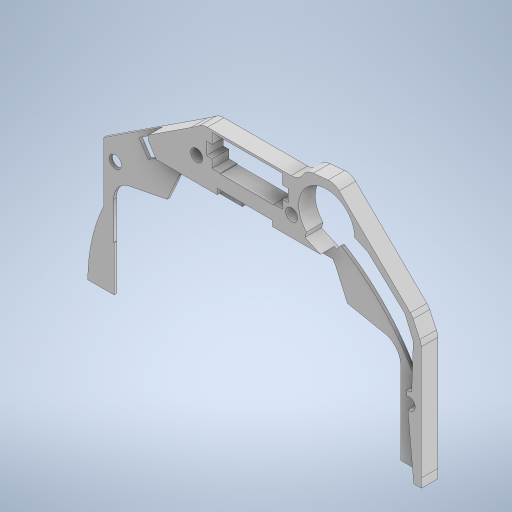
# Autodesk Inventor part: separator_right
Saved by Autodesk Inventor 2023.4 (Build 274418000, 418)
## iProperties
Created: 2024-02-02
Part Number: separator_right
Material: Generic
Document SubType Name: Modeling
Designer: aaron
Density: 1 g/cm^3
Appearance: Default
Author: aaron
Autodesk Inventor part; units mm, degrees
ref_plane "YZ Plane" through (0, 0, 0) normal (1, 0, 0) x (0, 1, 0)
ref_plane "XZ Plane" through (0, 0, 0) normal (0, 1, 0) x (-1, 0, 0)
ref_plane "XY Plane" through (0, 0, 0) normal (0, 0, 1) x (1, 0, 0)
sketch "Sketch1" plane through (0, 0, 0) normal (0, 0, 1) x (1, 0, 0)
  circle A0 centre (17.4431, 31.8315) radius 2.15
  circle A1 centre (-16.9982, 33.272) radius 2.15
  circle A2 centre (60.1072, -6.2422) radius 2.15
  circle A3 centre (-51.4779, 11.4956) radius 2.15
  arc A4 (-55.7008, -4.5478) -> (-61.4978, -30.6135) centre (0.0022, -30.6135) ccw
  line L0 (-61.4978, -30.6135) -> (-51.9975, -30.6135)
  line L1 (-51.9975, -30.6135) -> (-51.9975, -14.2185)
  line L2 (-51.9975, -14.2185) -> (-52.0975, -14.2185)
  line L3 (-52.0975, -14.2185) -> (-52.0975, -0.6135)
  arc A5 (-46.3779, 6.351) -> (-52.0975, -0.6135) centre (-44.9975, -0.6135) ccw
  line L4 (-46.3779, 6.351) -> (-32.7026, 9.0616)
  line L5 (-32.7026, 9.0616) -> (-28.4427, 18.6544)
  line L6 (-28.4427, 18.6544) -> (-27.4427, 20.3865)
  line L7 (-27.4427, 20.3865) -> (-5.4427, 20.3865)
  line L8 (-5.4427, 20.3865) -> (-5.4427, 23.8865)
  line L9 (-4.9427, 24.3865) -> (-5.4427, 23.8865)
  line L10 (-4.9427, 24.3865) -> (6.0573, 24.3865)
  line L11 (6.5573, 23.8865) -> (6.0573, 24.3865)
  line L12 (6.5573, 23.8865) -> (6.5573, 20.3865)
  line L13 (6.5573, 20.3865) -> (27.4471, 20.3865)
  line L14 (27.4471, 20.3865) -> (28.4471, 18.6544)
  line L15 (28.4471, 18.6544) -> (32.707, 9.0616)
  line L16 (32.707, 9.0616) -> (46.3823, 6.351)
  arc A6 (49.1747, 5.1308) -> (46.3823, 6.351) centre (45.0019, -0.6135) ccw
  line L17 (49.1747, 5.1308) -> (49.1159, 5.0499)
  arc A7 (52.0019, -0.6135) -> (49.1159, 5.0499) centre (45.0019, -0.6135) ccw
  line L18 (52.0019, -0.6135) -> (52.0019, -30.6135)
  line L19 (52.0019, -30.6135) -> (64.5022, -30.6135)
  arc A8 (64.5022, -30.6135) -> (64.4236, -27.4299) centre (0.0022, -30.6135) ccw
  line L20 (64.4236, -27.4299) -> (64.4236, 13.7348)
  arc A9 (64.4236, 13.7348) -> (63.951, 15.8567) centre (59.4236, 13.7348) ccw
  line L21 (63.951, 15.8567) -> (61.5154, 21.0535)
  arc A10 (61.5154, 21.0535) -> (60.4923, 22.4981) centre (56.988, 18.9315) ccw
  line L22 (60.4923, 22.4981) -> (34.6486, 47.8907)
  arc A11 (34.6486, 47.8907) -> (30.6723, 49.3019) centre (31.1444, 44.3242) ccw
  line L23 (30.6723, 49.3019) -> (25.3285, 48.7951)
  arc A12 (25.3285, 48.7951) -> (21.5187, 46.3993) centre (25.8005, 43.8174) ccw
  arc A13 (17.237, 43.9813) -> (21.5187, 46.3993) centre (17.237, 48.9813) ccw
  line L24 (-13.1205, 43.9813) -> (17.237, 43.9813)
  arc A14 (-13.1205, 43.9813) -> (-15.9723, 43.0882) centre (-13.1205, 38.9813) ccw
  line L25 (-15.9723, 43.0882) -> (-19.2592, 40.8057)
  line L26 (-55.7008, 17.024) -> (-19.2592, 40.8057)
  line L27 (-55.7008, -4.5478) -> (-55.7008, 17.024)
  line L28 (-8.3739, 31.6813) -> (-8.3739, 31.9813)
  line L29 (-8.3739, 31.9813) -> (-11.3739, 31.9813)
  line L30 (-11.3739, 31.9813) -> (-11.3739, 34.9813)
  line L31 (-11.3739, 34.9813) -> (-13.3739, 34.9813)
  line L32 (-13.3739, 34.9813) -> (-13.3739, 39.4813)
  line L33 (-13.3739, 39.4813) -> (-11.3739, 39.4813)
  line L34 (-11.3739, 39.4813) -> (-11.3739, 43.1813)
  line L35 (-11.3739, 43.1813) -> (14.1261, 43.1813)
  line L36 (14.1261, 43.1813) -> (14.1261, 39.4813)
  line L37 (14.1261, 39.4813) -> (16.1261, 39.4813)
  line L38 (16.1261, 39.4813) -> (16.1261, 34.9813)
  line L39 (16.1261, 34.9813) -> (14.1261, 34.9813)
  line L40 (14.1261, 34.9813) -> (14.1261, 31.9813)
  line L41 (14.1261, 31.9813) -> (11.1261, 31.9813)
  line L42 (11.1261, 31.9813) -> (11.1261, 31.6813)
  line L43 (11.1261, 31.6813) -> (-8.3739, 31.6813)
  arc A15 (30.18, 25.9182) -> (30.7743, 25.9371) centre (30.1536, 36.0569) ccw
  line L44 (30.18, 25.9182) -> (28.8398, 24.1662)
  line L45 (28.8398, 24.1662) -> (22.2728, 27.0821)
  line L46 (22.2728, 27.0821) -> (22.8312, 29.0443)
  arc A16 (40.2924, 36.0753) -> (22.8312, 29.0443) centre (30.1536, 36.0569) ccw
  line L47 (40.2924, 36.0753) -> (45.0482, 33.9636)
  line L48 (45.0482, 33.9636) -> (58.5651, 21.2864)
  line L49 (58.5651, 21.2864) -> (61.5673, 14.035)
  line L50 (61.5673, 14.035) -> (61.0022, -2.0891)
  line L51 (61.0022, -2.0891) -> (57.5886, -2.9772)
  arc A17 (57.5886, -2.9772) -> (30.7743, 25.9371) centre (-6.906, -35.8969) ccw
  line L52 (-39.547, 18.1923) -> (-42.9354, 23.3844)
  line L53 (-34.4498, 28.9221) -> (-42.9354, 23.3844)
  line L54 (-34.4498, 28.9221) -> (-31.0613, 23.73)
  line L55 (-31.0613, 23.73) -> (-39.547, 18.1923)
  point P0 (0, 0)
  constraints: 112 end point, 28 point on circle, 18 centre point
extrude "Extrusion1" add sketch "Sketch1" along normal blind 1
sketch "Sketch2" plane through (0, 0, 1) normal (0, 0, 1) x (1, 0, 0)
  line L0 (-19.2592, 40.8057) -> (-55.7008, 17.024) projected
  line L1 (-55.7008, 17.024) -> (-55.7008, -4.5478) projected
  arc A0 (-55.7008, -4.5478) -> (-61.4978, -30.6135) centre (0.0022, -30.6135) ccw projected
  line L2 (-61.4978, -30.6135) -> (-51.9975, -30.6135) projected
  line L3 (-51.9975, -30.6135) -> (-51.9975, -14.2185) projected
  line L4 (-51.9975, -14.2185) -> (-52.0975, -14.2185) projected
  line L5 (-52.0975, -14.2185) -> (-52.0975, -0.6135) projected
  arc A1 (-46.3779, 6.351) -> (-52.0975, -0.6135) centre (-44.9975, -0.6135) ccw projected
  line L6 (-46.3779, 6.351) -> (-32.7026, 9.0616) projected
  line L7 (-32.7026, 9.0616) -> (-28.4427, 18.6544) projected
  line L8 (-28.4427, 18.6544) -> (-27.4427, 20.3865) projected
  line L9 (-27.4427, 20.3865) -> (-5.4427, 20.3865) projected
  line L10 (-5.4427, 20.3865) -> (-5.4427, 23.8865) projected
  line L11 (-5.4427, 23.8865) -> (-4.9427, 24.3865) projected
  line L12 (-4.9427, 24.3865) -> (6.0573, 24.3865) projected
  line L13 (6.0573, 24.3865) -> (6.5573, 23.8865) projected
  line L14 (6.5573, 23.8865) -> (6.5573, 20.3865) projected
  line L15 (6.5573, 20.3865) -> (27.4471, 20.3865) projected
  line L16 (27.4471, 20.3865) -> (28.4471, 18.6544) projected
  line L17 (28.4471, 18.6544) -> (32.707, 9.0616) projected
  line L18 (32.707, 9.0616) -> (46.3823, 6.351) projected
  arc A2 (49.1747, 5.1308) -> (46.3823, 6.351) centre (45.0019, -0.6135) ccw projected
  line L19 (49.1747, 5.1308) -> (49.1159, 5.0499) projected
  arc A3 (52.0019, -0.6135) -> (49.1159, 5.0499) centre (45.0019, -0.6135) ccw projected
  line L20 (52.0019, -0.6135) -> (52.0019, -30.6135) projected
  line L21 (52.0019, -30.6135) -> (64.5022, -30.6135) projected
  arc A4 (64.5022, -30.6135) -> (64.4236, -27.4299) centre (0.0022, -30.6135) ccw projected
  line L22 (64.4236, -27.4299) -> (64.4236, 13.7348) projected
  arc A5 (64.4236, 13.7348) -> (63.951, 15.8567) centre (59.4236, 13.7348) ccw projected
  line L23 (63.951, 15.8567) -> (61.5154, 21.0535) projected
  arc A6 (61.5154, 21.0535) -> (60.4923, 22.4981) centre (56.988, 18.9315) ccw projected
  line L24 (60.4923, 22.4981) -> (34.6486, 47.8907) projected
  arc A7 (34.6486, 47.8907) -> (30.6723, 49.3019) centre (31.1444, 44.3242) ccw projected
  line L25 (30.6723, 49.3019) -> (25.3285, 48.7951) projected
  arc A8 (25.3285, 48.7951) -> (21.5187, 46.3993) centre (25.8005, 43.8174) ccw projected
  arc A9 (17.237, 43.9813) -> (21.5187, 46.3993) centre (17.237, 48.9813) ccw projected
  line L26 (17.237, 43.9813) -> (-13.1205, 43.9813) projected
  arc A10 (-13.1205, 43.9813) -> (-15.9723, 43.0882) centre (-13.1205, 38.9813) ccw projected
  line L27 (-15.9723, 43.0882) -> (-19.2592, 40.8057) projected
  circle A11 centre (60.1072, -6.2422) radius 2.15 projected
  circle A12 centre (-51.4779, 11.4956) radius 2.15 projected
  circle A13 centre (17.4431, 31.8315) radius 2.15 projected
  circle A14 centre (-16.9982, 33.272) radius 2.15 projected
  line L28 (-34.4498, 28.9221) -> (-31.0613, 23.73) projected
  line L29 (-31.0613, 23.73) -> (-39.547, 18.1923) projected
  line L30 (-39.547, 18.1923) -> (-42.9354, 23.3844) projected
  line L31 (-42.9354, 23.3844) -> (-34.4498, 28.9221) projected
  line L32 (40.2924, 36.0753) -> (45.0482, 33.9636) projected
  line L33 (45.0482, 33.9636) -> (58.5651, 21.2864) projected
  line L34 (58.5651, 21.2864) -> (61.5673, 14.035) projected
  line L35 (61.5673, 14.035) -> (61.0022, -2.0891) projected
  line L36 (61.0022, -2.0891) -> (57.5886, -2.9772) projected
  arc A15 (57.5886, -2.9772) -> (30.7743, 25.9371) centre (-6.906, -35.8969) ccw projected
  arc A16 (30.18, 25.9182) -> (30.7743, 25.9371) centre (30.1536, 36.0569) ccw projected
  line L37 (30.18, 25.9182) -> (28.8398, 24.1662) projected
  line L38 (28.8398, 24.1662) -> (22.2728, 27.0821) projected
  line L39 (22.2728, 27.0821) -> (22.8312, 29.0443) projected
  arc A17 (40.2924, 36.0753) -> (22.8312, 29.0443) centre (30.1536, 36.0569) ccw projected
  line L40 (11.1261, 31.6813) -> (-8.3739, 31.6813) projected
  line L41 (-8.3739, 31.6813) -> (-8.3739, 31.9813) projected
  line L42 (-8.3739, 31.9813) -> (-11.3739, 31.9813) projected
  line L43 (-11.3739, 31.9813) -> (-11.3739, 34.9813) projected
  line L44 (-11.3739, 34.9813) -> (-13.3739, 34.9813) projected
  line L45 (-13.3739, 34.9813) -> (-13.3739, 39.4813) projected
  line L46 (-13.3739, 39.4813) -> (-11.3739, 39.4813) projected
  line L47 (-11.3739, 39.4813) -> (-11.3739, 43.1813) projected
  line L48 (-11.3739, 43.1813) -> (14.1261, 43.1813) projected
  line L49 (14.1261, 43.1813) -> (14.1261, 39.4813) projected
  line L50 (14.1261, 39.4813) -> (16.1261, 39.4813) projected
  line L51 (16.1261, 39.4813) -> (16.1261, 34.9813) projected
  line L52 (16.1261, 34.9813) -> (14.1261, 34.9813) projected
  line L53 (14.1261, 34.9813) -> (14.1261, 31.9813) projected
  line L54 (14.1261, 31.9813) -> (11.1261, 31.9813) projected
  line L55 (11.1261, 31.9813) -> (11.1261, 31.6813) projected
  arc A18 (-54.3404, 17.9118) -> (-55.7008, 15.3995) centre (-52.7008, 15.3995) ccw
  line L56 (-45.7894, 6.3415) -> (-45.7894, 6.4676)
  line L57 (-45.7894, 6.4676) -> (-46.3779, 6.351)
  circle A19 centre (-51.4779, 11.4956) radius 1.7
  line L58 (-55.7008, 9.3609) -> (-55.7008, 15.3995)
  arc A20 (-46.3779, 6.351) -> (-48.8352, 5.3599) centre (-44.9975, -0.6135) ccw
  arc A21 (-55.7008, 9.3609) -> (-54.3502, 6.855) centre (-52.7008, 9.3609) ccw
  line L59 (-52.1062, 5.378) -> (-54.3502, 6.855)
  arc A22 (-52.1062, 5.378) -> (-48.8352, 5.3599) centre (-50.4568, 7.8839) ccw
  line L60 (-33.0873, 8.1945) -> (-45.7894, 6.3415)
  line L61 (-31.6168, 24.581) -> (-9.5427, 24.581)
  line L62 (-5.5427, 20.3865) -> (-27.4423, 20.3865)
  line L63 (-9.5427, 24.581) -> (-9.5427, 26.581)
  line L64 (-4.9841, 24.4865) -> (-5.5427, 23.9279)
  line L65 (6.0988, 24.4865) -> (-4.9841, 24.4865)
  line L66 (10.4573, 26.581) -> (-9.5427, 26.581)
  line L67 (-5.5427, 23.9279) -> (-5.5427, 20.3865)
  line L68 (6.6573, 23.9279) -> (6.0988, 24.4865)
  line L69 (6.6573, 20.3865) -> (6.6573, 23.9279)
  line L70 (10.4573, 24.581) -> (10.4573, 26.581)
  line L71 (27.4474, 20.3865) -> (6.6573, 20.3865)
  line L72 (28.4474, 18.6544) -> (27.4474, 20.3865)
  line L73 (10.4573, 24.581) -> (33.7945, 24.581)
  arc A23 (33.0924, 8.1945) -> (25.5025, 13.5538) centre (0.0025, -30.6135) ccw
  line L74 (45.7945, 12.581) -> (33.7945, 24.581)
  line L75 (45.7945, 12.581) -> (45.7945, 6.3415)
  line L76 (45.7945, 6.3415) -> (33.0924, 8.1945)
  line L77 (25.5025, 13.5538) -> (28.4474, 18.6544)
  line L78 (-54.3404, 17.9118) -> (-34.4498, 30.8924)
  arc A24 (-25.4975, 13.5538) -> (-33.0873, 8.1945) centre (0.0025, -30.6135) ccw
  line L79 (-28.4423, 18.6544) -> (-25.4975, 13.5538)
  line L80 (-42.9354, 23.3844) -> (-39.547, 18.1923)
  line L81 (-27.4423, 20.3865) -> (-28.4423, 18.6544)
  line L82 (-39.547, 18.1923) -> (-31.0613, 23.73)
  line L83 (-31.0613, 23.73) -> (-31.6168, 24.581)
  line L84 (-34.4498, 28.9221) -> (-42.9354, 23.3844)
  line L85 (-34.4498, 30.8924) -> (-34.4498, 28.9221)
  line L86 (-34.4498, 28.9221) -> (-31.0613, 23.73) projected
  line L87 (-32.7555, 26.3261) -> (-12.0803, 38.0318)
  line L88 (13.5764, 37.2313) -> (24.9592, 37.4875)
  line L89 (58.5651, 2.815) -> (62.2572, -35.8969)
  point P0 (0, 0)
  point P1 (27.9056, 24.581)
  point P2 (59.0805, -2.5891)
  point P3 (59.2413, -4.2743)
  point P4 (59.6288, -8.3383)
  point P5 (61.7533, -30.6135)
  constraints: 66 end point, 12 point on circle, 7 centre point, 1 midpoint
extrude "Extrusion2" add sketch "Sketch2" along normal blind 5 contours L27 A10 L26 A9 A8 L25 A7 L24 A6 L23 A5 L22 A4 L21 L89 A11 L36 L35 L34 L33 L32 A17 L88 L51 L50 L49 L48 L47 L46 L45 L87 A14 L28 L85 L0 | L87 A14 L45 L44 L43 L42 L41 L40 L55 L54 L53 L52 L51 L88 A17 L39 L38 L73 L70 L66 L63 L61 L28
body "Solid1"
